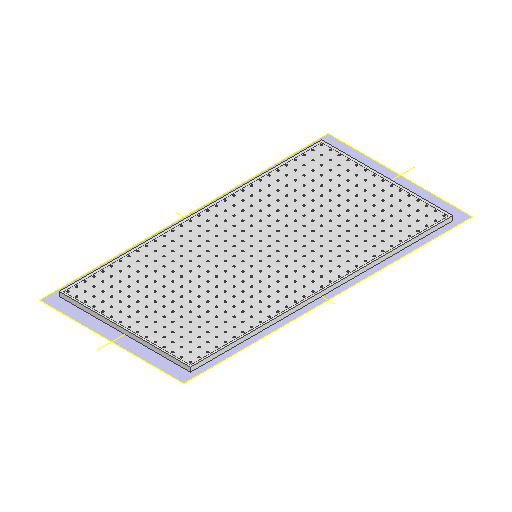
# Autodesk Inventor part: 판넬
Saved by Autodesk Inventor 2027 (Build 310192000, 192)
## iProperties
Created: 2026-09-29
Part Number: 판넬
Material: 일반
Document SubType Name: Modeling
Designer: User
Density: 1 g/cm^3
Appearance: 기본값
Author: User
Autodesk Inventor part; units mm, degrees
ref_plane "YZ 평면_우측면도" through (0, 0, 0) normal (1, 0, 0) x (0, 1, 0)
ref_plane "XZ 평면_평면도" through (0, 0, 0) normal (0, 1, 0) x (-1, 0, 0)
ref_plane "XY 평면_정면도" through (0, 0, 0) normal (0, 0, 1) x (1, 0, 0)
sketch "스케치1" plane through (0, 0, 0) normal (0, 1, 0) x (-1, 0, 0)
  line L0 (150, -300) -> (-150, -300)
  line L1 (-150, -300) -> (-150, 300)
  line L2 (-150, 300) -> (150, 300)
  line L3 (150, 300) -> (150, -300)
  line L4 (150, -300) -> (-150, 300) construction
  line L5 (-150, -300) -> (150, 300) construction
  line L6 (-150, 300) -> (-140, 300)
  line L7 (-140, 300) -> (-140, 290) construction
  line L8 (-140, 290) -> (-150, 290) construction
  line L9 (-150, 290) -> (-150, 300)
  circle A0 centre (-140, 290) radius 2
  circle A1 centre (-120, 290) radius 2
  circle A2 centre (-100, 290) radius 2
  circle A3 centre (-80, 290) radius 2
  circle A4 centre (-60, 290) radius 2
  circle A5 centre (-40, 290) radius 2
  circle A6 centre (-20, 290) radius 2
  circle A7 centre (0, 290) radius 2
  circle A8 centre (20, 290) radius 2
  circle A9 centre (40, 290) radius 2
  circle A10 centre (60, 290) radius 2
  circle A11 centre (80, 290) radius 2
  circle A12 centre (100, 290) radius 2
  circle A13 centre (120, 290) radius 2
  circle A14 centre (140, 290) radius 2
  circle A15 centre (-140, 270) radius 2
  circle A16 centre (-120, 270) radius 2
  circle A17 centre (-100, 270) radius 2
  circle A18 centre (-80, 270) radius 2
  circle A19 centre (-60, 270) radius 2
  circle A20 centre (-40, 270) radius 2
  circle A21 centre (-20, 270) radius 2
  circle A22 centre (0, 270) radius 2
  circle A23 centre (20, 270) radius 2
  circle A24 centre (40, 270) radius 2
  circle A25 centre (60, 270) radius 2
  circle A26 centre (80, 270) radius 2
  circle A27 centre (100, 270) radius 2
  circle A28 centre (120, 270) radius 2
  circle A29 centre (140, 270) radius 2
  circle A30 centre (-140, 250) radius 2
  circle A31 centre (-120, 250) radius 2
  circle A32 centre (-100, 250) radius 2
  circle A33 centre (-80, 250) radius 2
  circle A34 centre (-60, 250) radius 2
  circle A35 centre (-40, 250) radius 2
  circle A36 centre (-20, 250) radius 2
  circle A37 centre (0, 250) radius 2
  circle A38 centre (20, 250) radius 2
  circle A39 centre (40, 250) radius 2
  circle A40 centre (60, 250) radius 2
  circle A41 centre (80, 250) radius 2
  circle A42 centre (100, 250) radius 2
  circle A43 centre (120, 250) radius 2
  circle A44 centre (140, 250) radius 2
  circle A45 centre (-140, 230) radius 2
  circle A46 centre (-120, 230) radius 2
  circle A47 centre (-100, 230) radius 2
  circle A48 centre (-80, 230) radius 2
  circle A49 centre (-60, 230) radius 2
  circle A50 centre (-40, 230) radius 2
  circle A51 centre (-20, 230) radius 2
  circle A52 centre (0, 230) radius 2
  circle A53 centre (20, 230) radius 2
  circle A54 centre (40, 230) radius 2
  circle A55 centre (60, 230) radius 2
  circle A56 centre (80, 230) radius 2
  circle A57 centre (100, 230) radius 2
  circle A58 centre (120, 230) radius 2
  circle A59 centre (140, 230) radius 2
  circle A60 centre (-140, 210) radius 2
  circle A61 centre (-120, 210) radius 2
  circle A62 centre (-100, 210) radius 2
  circle A63 centre (-80, 210) radius 2
  circle A64 centre (-60, 210) radius 2
  circle A65 centre (-40, 210) radius 2
  circle A66 centre (-20, 210) radius 2
  circle A67 centre (0, 210) radius 2
  circle A68 centre (20, 210) radius 2
  circle A69 centre (40, 210) radius 2
  circle A70 centre (60, 210) radius 2
  circle A71 centre (80, 210) radius 2
  circle A72 centre (100, 210) radius 2
  circle A73 centre (120, 210) radius 2
  circle A74 centre (140, 210) radius 2
  circle A75 centre (-140, 190) radius 2
  circle A76 centre (-120, 190) radius 2
  circle A77 centre (-100, 190) radius 2
  circle A78 centre (-80, 190) radius 2
  circle A79 centre (-60, 190) radius 2
  circle A80 centre (-40, 190) radius 2
  circle A81 centre (-20, 190) radius 2
  circle A82 centre (0, 190) radius 2
  circle A83 centre (20, 190) radius 2
  circle A84 centre (40, 190) radius 2
  circle A85 centre (60, 190) radius 2
  circle A86 centre (80, 190) radius 2
  circle A87 centre (100, 190) radius 2
  circle A88 centre (120, 190) radius 2
  circle A89 centre (140, 190) radius 2
  circle A90 centre (-140, 170) radius 2
  circle A91 centre (-120, 170) radius 2
  circle A92 centre (-100, 170) radius 2
  circle A93 centre (-80, 170) radius 2
  circle A94 centre (-60, 170) radius 2
  circle A95 centre (-40, 170) radius 2
  circle A96 centre (-20, 170) radius 2
  circle A97 centre (0, 170) radius 2
  circle A98 centre (20, 170) radius 2
  circle A99 centre (40, 170) radius 2
  circle A100 centre (60, 170) radius 2
  circle A101 centre (80, 170) radius 2
  circle A102 centre (100, 170) radius 2
  circle A103 centre (120, 170) radius 2
  circle A104 centre (140, 170) radius 2
  circle A105 centre (-140, 150) radius 2
  circle A106 centre (-120, 150) radius 2
  circle A107 centre (-100, 150) radius 2
  circle A108 centre (-80, 150) radius 2
  circle A109 centre (-60, 150) radius 2
  circle A110 centre (-40, 150) radius 2
  circle A111 centre (-20, 150) radius 2
  circle A112 centre (0, 150) radius 2
  circle A113 centre (20, 150) radius 2
  circle A114 centre (40, 150) radius 2
  circle A115 centre (60, 150) radius 2
  circle A116 centre (80, 150) radius 2
  circle A117 centre (100, 150) radius 2
  circle A118 centre (120, 150) radius 2
  circle A119 centre (140, 150) radius 2
  circle A120 centre (-140, 130) radius 2
  circle A121 centre (-120, 130) radius 2
  circle A122 centre (-100, 130) radius 2
  circle A123 centre (-80, 130) radius 2
  circle A124 centre (-60, 130) radius 2
  circle A125 centre (-40, 130) radius 2
  circle A126 centre (-20, 130) radius 2
  circle A127 centre (0, 130) radius 2
  circle A128 centre (20, 130) radius 2
  circle A129 centre (40, 130) radius 2
  circle A130 centre (60, 130) radius 2
  circle A131 centre (80, 130) radius 2
  circle A132 centre (100, 130) radius 2
  circle A133 centre (120, 130) radius 2
  circle A134 centre (140, 130) radius 2
  circle A135 centre (-140, 110) radius 2
  circle A136 centre (-120, 110) radius 2
  circle A137 centre (-100, 110) radius 2
  circle A138 centre (-80, 110) radius 2
  circle A139 centre (-60, 110) radius 2
  circle A140 centre (-40, 110) radius 2
  circle A141 centre (-20, 110) radius 2
  circle A142 centre (0, 110) radius 2
  circle A143 centre (20, 110) radius 2
  circle A144 centre (40, 110) radius 2
  circle A145 centre (60, 110) radius 2
  circle A146 centre (80, 110) radius 2
  circle A147 centre (100, 110) radius 2
  circle A148 centre (120, 110) radius 2
  circle A149 centre (140, 110) radius 2
  circle A150 centre (-140, 90) radius 2
  circle A151 centre (-120, 90) radius 2
  circle A152 centre (-100, 90) radius 2
  circle A153 centre (-80, 90) radius 2
  circle A154 centre (-60, 90) radius 2
  circle A155 centre (-40, 90) radius 2
  circle A156 centre (-20, 90) radius 2
  circle A157 centre (0, 90) radius 2
  circle A158 centre (20, 90) radius 2
  circle A159 centre (40, 90) radius 2
  circle A160 centre (60, 90) radius 2
  circle A161 centre (80, 90) radius 2
  circle A162 centre (100, 90) radius 2
  circle A163 centre (120, 90) radius 2
  circle A164 centre (140, 90) radius 2
  circle A165 centre (-140, 70) radius 2
  circle A166 centre (-120, 70) radius 2
  circle A167 centre (-100, 70) radius 2
  circle A168 centre (-80, 70) radius 2
  circle A169 centre (-60, 70) radius 2
  circle A170 centre (-40, 70) radius 2
  circle A171 centre (-20, 70) radius 2
  circle A172 centre (0, 70) radius 2
  circle A173 centre (20, 70) radius 2
  circle A174 centre (40, 70) radius 2
  circle A175 centre (60, 70) radius 2
  circle A176 centre (80, 70) radius 2
  circle A177 centre (100, 70) radius 2
  circle A178 centre (120, 70) radius 2
  circle A179 centre (140, 70) radius 2
  circle A180 centre (-140, 50) radius 2
  circle A181 centre (-120, 50) radius 2
  circle A182 centre (-100, 50) radius 2
  circle A183 centre (-80, 50) radius 2
  circle A184 centre (-60, 50) radius 2
  circle A185 centre (-40, 50) radius 2
  circle A186 centre (-20, 50) radius 2
  circle A187 centre (0, 50) radius 2
  circle A188 centre (20, 50) radius 2
  circle A189 centre (40, 50) radius 2
  circle A190 centre (60, 50) radius 2
  circle A191 centre (80, 50) radius 2
  circle A192 centre (100, 50) radius 2
  circle A193 centre (120, 50) radius 2
  circle A194 centre (140, 50) radius 2
  circle A195 centre (-140, 30) radius 2
  circle A196 centre (-120, 30) radius 2
  circle A197 centre (-100, 30) radius 2
  circle A198 centre (-80, 30) radius 2
  circle A199 centre (-60, 30) radius 2
  circle A200 centre (-40, 30) radius 2
  circle A201 centre (-20, 30) radius 2
  circle A202 centre (0, 30) radius 2
  circle A203 centre (20, 30) radius 2
  circle A204 centre (40, 30) radius 2
  circle A205 centre (60, 30) radius 2
  circle A206 centre (80, 30) radius 2
  circle A207 centre (100, 30) radius 2
  circle A208 centre (120, 30) radius 2
  circle A209 centre (140, 30) radius 2
  circle A210 centre (-140, 10) radius 2
  circle A211 centre (-120, 10) radius 2
  circle A212 centre (-100, 10) radius 2
  circle A213 centre (-80, 10) radius 2
  circle A214 centre (-60, 10) radius 2
  circle A215 centre (-40, 10) radius 2
  circle A216 centre (-20, 10) radius 2
  circle A217 centre (0, 10) radius 2
  circle A218 centre (20, 10) radius 2
  circle A219 centre (40, 10) radius 2
  circle A220 centre (60, 10) radius 2
  circle A221 centre (80, 10) radius 2
  circle A222 centre (100, 10) radius 2
  circle A223 centre (120, 10) radius 2
  circle A224 centre (140, 10) radius 2
  circle A225 centre (-140, -10) radius 2
  circle A226 centre (-120, -10) radius 2
  circle A227 centre (-100, -10) radius 2
  circle A228 centre (-80, -10) radius 2
  circle A229 centre (-60, -10) radius 2
  circle A230 centre (-40, -10) radius 2
  circle A231 centre (-20, -10) radius 2
  circle A232 centre (0, -10) radius 2
  circle A233 centre (20, -10) radius 2
  circle A234 centre (40, -10) radius 2
  circle A235 centre (60, -10) radius 2
  circle A236 centre (80, -10) radius 2
  circle A237 centre (100, -10) radius 2
  circle A238 centre (120, -10) radius 2
  circle A239 centre (140, -10) radius 2
  circle A240 centre (-140, -30) radius 2
  circle A241 centre (-120, -30) radius 2
  circle A242 centre (-100, -30) radius 2
  circle A243 centre (-80, -30) radius 2
  circle A244 centre (-60, -30) radius 2
  circle A245 centre (-40, -30) radius 2
  circle A246 centre (-20, -30) radius 2
  circle A247 centre (0, -30) radius 2
  circle A248 centre (20, -30) radius 2
  circle A249 centre (40, -30) radius 2
  circle A250 centre (60, -30) radius 2
  circle A251 centre (80, -30) radius 2
  circle A252 centre (100, -30) radius 2
  circle A253 centre (120, -30) radius 2
  circle A254 centre (140, -30) radius 2
  circle A255 centre (-140, -50) radius 2
  circle A256 centre (-120, -50) radius 2
  circle A257 centre (-100, -50) radius 2
  circle A258 centre (-80, -50) radius 2
  circle A259 centre (-60, -50) radius 2
  circle A260 centre (-40, -50) radius 2
  circle A261 centre (-20, -50) radius 2
  circle A262 centre (0, -50) radius 2
  circle A263 centre (20, -50) radius 2
  circle A264 centre (40, -50) radius 2
  circle A265 centre (60, -50) radius 2
  circle A266 centre (80, -50) radius 2
  circle A267 centre (100, -50) radius 2
  circle A268 centre (120, -50) radius 2
  circle A269 centre (140, -50) radius 2
  circle A270 centre (-140, -70) radius 2
  circle A271 centre (-120, -70) radius 2
  circle A272 centre (-100, -70) radius 2
  circle A273 centre (-80, -70) radius 2
  circle A274 centre (-60, -70) radius 2
  circle A275 centre (-40, -70) radius 2
  circle A276 centre (-20, -70) radius 2
  circle A277 centre (0, -70) radius 2
  circle A278 centre (20, -70) radius 2
  circle A279 centre (40, -70) radius 2
  circle A280 centre (60, -70) radius 2
  circle A281 centre (80, -70) radius 2
  circle A282 centre (100, -70) radius 2
  circle A283 centre (120, -70) radius 2
  circle A284 centre (140, -70) radius 2
  circle A285 centre (-140, -90) radius 2
  circle A286 centre (-120, -90) radius 2
  circle A287 centre (-100, -90) radius 2
  circle A288 centre (-80, -90) radius 2
  circle A289 centre (-60, -90) radius 2
  circle A290 centre (-40, -90) radius 2
  circle A291 centre (-20, -90) radius 2
  circle A292 centre (0, -90) radius 2
  circle A293 centre (20, -90) radius 2
  circle A294 centre (40, -90) radius 2
  circle A295 centre (60, -90) radius 2
  circle A296 centre (80, -90) radius 2
  circle A297 centre (100, -90) radius 2
  circle A298 centre (120, -90) radius 2
  circle A299 centre (140, -90) radius 2
  circle A300 centre (-140, -110) radius 2
  circle A301 centre (-120, -110) radius 2
  circle A302 centre (-100, -110) radius 2
  circle A303 centre (-80, -110) radius 2
  circle A304 centre (-60, -110) radius 2
  circle A305 centre (-40, -110) radius 2
  circle A306 centre (-20, -110) radius 2
  circle A307 centre (0, -110) radius 2
  circle A308 centre (20, -110) radius 2
  circle A309 centre (40, -110) radius 2
  circle A310 centre (60, -110) radius 2
  circle A311 centre (80, -110) radius 2
  circle A312 centre (100, -110) radius 2
  circle A313 centre (120, -110) radius 2
  circle A314 centre (140, -110) radius 2
  circle A315 centre (-140, -130) radius 2
  circle A316 centre (-120, -130) radius 2
  circle A317 centre (-100, -130) radius 2
  circle A318 centre (-80, -130) radius 2
  circle A319 centre (-60, -130) radius 2
  circle A320 centre (-40, -130) radius 2
  circle A321 centre (-20, -130) radius 2
  circle A322 centre (0, -130) radius 2
  circle A323 centre (20, -130) radius 2
  circle A324 centre (40, -130) radius 2
  circle A325 centre (60, -130) radius 2
  circle A326 centre (80, -130) radius 2
  circle A327 centre (100, -130) radius 2
  circle A328 centre (120, -130) radius 2
  circle A329 centre (140, -130) radius 2
  circle A330 centre (-140, -150) radius 2
  circle A331 centre (-120, -150) radius 2
  circle A332 centre (-100, -150) radius 2
  circle A333 centre (-80, -150) radius 2
  circle A334 centre (-60, -150) radius 2
  circle A335 centre (-40, -150) radius 2
  circle A336 centre (-20, -150) radius 2
  circle A337 centre (0, -150) radius 2
  circle A338 centre (20, -150) radius 2
  circle A339 centre (40, -150) radius 2
  circle A340 centre (60, -150) radius 2
  circle A341 centre (80, -150) radius 2
  circle A342 centre (100, -150) radius 2
  circle A343 centre (120, -150) radius 2
  circle A344 centre (140, -150) radius 2
  circle A345 centre (-140, -170) radius 2
  circle A346 centre (-120, -170) radius 2
  circle A347 centre (-100, -170) radius 2
  circle A348 centre (-80, -170) radius 2
  circle A349 centre (-60, -170) radius 2
  circle A350 centre (-40, -170) radius 2
  circle A351 centre (-20, -170) radius 2
  circle A352 centre (0, -170) radius 2
  circle A353 centre (20, -170) radius 2
  circle A354 centre (40, -170) radius 2
  circle A355 centre (60, -170) radius 2
  circle A356 centre (80, -170) radius 2
  circle A357 centre (100, -170) radius 2
  circle A358 centre (120, -170) radius 2
  circle A359 centre (140, -170) radius 2
  circle A360 centre (-140, -190) radius 2
  circle A361 centre (-120, -190) radius 2
  circle A362 centre (-100, -190) radius 2
  circle A363 centre (-80, -190) radius 2
  circle A364 centre (-60, -190) radius 2
  circle A365 centre (-40, -190) radius 2
  circle A366 centre (-20, -190) radius 2
  circle A367 centre (0, -190) radius 2
  circle A368 centre (20, -190) radius 2
  circle A369 centre (40, -190) radius 2
  circle A370 centre (60, -190) radius 2
  circle A371 centre (80, -190) radius 2
  circle A372 centre (100, -190) radius 2
  circle A373 centre (120, -190) radius 2
  circle A374 centre (140, -190) radius 2
  circle A375 centre (-140, -210) radius 2
  circle A376 centre (-120, -210) radius 2
  circle A377 centre (-100, -210) radius 2
  circle A378 centre (-80, -210) radius 2
  circle A379 centre (-60, -210) radius 2
  circle A380 centre (-40, -210) radius 2
  circle A381 centre (-20, -210) radius 2
  circle A382 centre (0, -210) radius 2
  circle A383 centre (20, -210) radius 2
  circle A384 centre (40, -210) radius 2
  circle A385 centre (60, -210) radius 2
  circle A386 centre (80, -210) radius 2
  circle A387 centre (100, -210) radius 2
  circle A388 centre (120, -210) radius 2
  circle A389 centre (140, -210) radius 2
  circle A390 centre (-140, -230) radius 2
  circle A391 centre (-120, -230) radius 2
  circle A392 centre (-100, -230) radius 2
  circle A393 centre (-80, -230) radius 2
  circle A394 centre (-60, -230) radius 2
  circle A395 centre (-40, -230) radius 2
  circle A396 centre (-20, -230) radius 2
  circle A397 centre (0, -230) radius 2
  circle A398 centre (20, -230) radius 2
  circle A399 centre (40, -230) radius 2
  circle A400 centre (60, -230) radius 2
  circle A401 centre (80, -230) radius 2
  circle A402 centre (100, -230) radius 2
  circle A403 centre (120, -230) radius 2
  circle A404 centre (140, -230) radius 2
  circle A405 centre (-140, -250) radius 2
  circle A406 centre (-120, -250) radius 2
  circle A407 centre (-100, -250) radius 2
  circle A408 centre (-80, -250) radius 2
  circle A409 centre (-60, -250) radius 2
  circle A410 centre (-40, -250) radius 2
  circle A411 centre (-20, -250) radius 2
  circle A412 centre (0, -250) radius 2
  circle A413 centre (20, -250) radius 2
  circle A414 centre (40, -250) radius 2
  circle A415 centre (60, -250) radius 2
  circle A416 centre (80, -250) radius 2
  circle A417 centre (100, -250) radius 2
  circle A418 centre (120, -250) radius 2
  circle A419 centre (140, -250) radius 2
  circle A420 centre (-140, -270) radius 2
  circle A421 centre (-120, -270) radius 2
  circle A422 centre (-100, -270) radius 2
  circle A423 centre (-80, -270) radius 2
  circle A424 centre (-60, -270) radius 2
  circle A425 centre (-40, -270) radius 2
  circle A426 centre (-20, -270) radius 2
  circle A427 centre (0, -270) radius 2
  circle A428 centre (20, -270) radius 2
  circle A429 centre (40, -270) radius 2
  circle A430 centre (60, -270) radius 2
  circle A431 centre (80, -270) radius 2
  circle A432 centre (100, -270) radius 2
  circle A433 centre (120, -270) radius 2
  circle A434 centre (140, -270) radius 2
  circle A435 centre (-140, -290) radius 2
  circle A436 centre (-120, -290) radius 2
  circle A437 centre (-100, -290) radius 2
  circle A438 centre (-80, -290) radius 2
  circle A439 centre (-60, -290) radius 2
  circle A440 centre (-40, -290) radius 2
  circle A441 centre (-20, -290) radius 2
  circle A442 centre (0, -290) radius 2
  circle A443 centre (20, -290) radius 2
  circle A444 centre (40, -290) radius 2
  circle A445 centre (60, -290) radius 2
  circle A446 centre (80, -290) radius 2
  circle A447 centre (100, -290) radius 2
  circle A448 centre (120, -290) radius 2
  circle A449 centre (140, -290) radius 2
  point P0 (0, 0)
  dimension "d0" = 300
  dimension "d1" = 600
  dimension "d2" = 10
  dimension "d3" = 10
  dimension "d4" = 4
  dimension "d7" = 20
  dimension "d10" = 20
  constraints: 450 centre point, 20 end point, 4 parallel, 3 horizontal, 2 midpoint, 2 perpendicular, 1 coincident, 1 vertical, 898 other
  measures "d0" distance of L1.end L2.end
  measures "d1" distance of L0.end L1.end
  measures "d2" distance of L7.end L8.end
  measures "d3" distance of L6.end L7.end
  measures "d4" diameter of A0
  measures "d7" distance of A0.centre A1.centre
  measures "d10" distance of A0.centre A15.centre
extrude "돌출1" add sketch "스케치1" along normal blind 10
ref_plane "작업 평면1" through (0, 0, 0) normal (0, -1, 0) x (1, 0, 0)
sketch "스케치3" plane through (0, 0, 0) normal (0, -1, 0) x (1, 0, 0)
  line L0 (150, -300) -> (-150, -300) projected
  line L1 (150, 300) -> (150, -300) projected
  line L2 (-150, 300) -> (150, 300) projected
  line L3 (-150, -300) -> (-150, 300) projected
  line L4 (-145, -295) -> (145, -295)
  line L5 (145, -295) -> (145, 295)
  line L6 (145, 295) -> (-145, 295)
  line L7 (-145, 295) -> (-145, -295)
  point P0 (0, 0)
  dimension "d16" = 5
  constraints: 8 end point, 3 other
  measures "d16" distance between parallel lines of L0 L4
extrude "돌출2" cut sketch "스케치3" against normal blind 9 contours L7 L6 L5 L4
